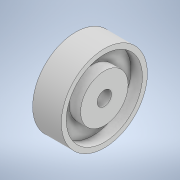
# Autodesk Inventor part: 711145
Saved by Autodesk Inventor 2022 (Build 260153000, 153)
## iProperties
Created: 2021-10-22
Part Number: 711145
Material: Типовые
Document SubType Name: Modeling
Designer: RaNSiD
Density: 1 g/cm^3
Appearance: По умолчанию
Author: RaNSiD
Autodesk Inventor part; units mm, degrees
ref_plane "YZ Plane" through (0, 0, 0) normal (1, 0, 0) x (0, 1, 0)
ref_plane "XZ Plane" through (0, 0, 0) normal (0, 1, 0) x (-1, 0, 0)
ref_plane "XY Plane" through (0, 0, 0) normal (0, 0, 1) x (1, 0, 0)
sketch "Эскиз1" plane through (0, 0, 0) normal (0, 0, 1) x (1, 0, 0)
  line L0 (0, 0) -> (20, 0)
  line L1 (20, 0) -> (20, 30)
  line L2 (20, 30) -> (0, 30)
  line L3 (0, 30) -> (0, 0)
  dimension "d0" = 20
  dimension "d1" = 30
  constraints: 8 end point, 2 parallel, 1 horizontal, 1 perpendicular
  measures "d0" distance of L2.end L1.end
  measures "d1" distance of L1.end L0.end
revolve "Вращение1" add sketch "Эскиз1" angle 360 about axis through (0, 0, 0) along (1, 0, 0)
sketch "Эскиз2" plane through (0, 0, 0) normal (0, 0, 1) x (1, 0, 0)
  line L0 (0, -30) -> (0, 30) projected
  line L1 (0, 15.0882) -> (0, 28)
  line L2 (0, 28) -> (4, 26.5441)
  line L3 (4, 26.5441) -> (4, 16.5441)
  line L4 (4, 16.5441) -> (0, 15.0882)
  line L5 (20, -30) -> (20, 30) projected
  line L6 (20, 26.5441) -> (12, 26.5441)
  line L7 (12, 26.5441) -> (12, 16.5441)
  line L8 (12, 16.5441) -> (20, 16.5441)
  line L9 (20, 16.5441) -> (20, 26.5441)
  line L10 (0, 0) -> (20, 0)
  line L11 (20, 0) -> (20, 5)
  line L12 (20, 5) -> (0, 5)
  line L13 (0, 5) -> (0, 0)
  point P0 (0, 5)
  dimension "d3" = 10
  dimension "d4" = 8
  dimension "d5" = 10
  dimension "d6" = 2
  dimension "d7" = 70
  dimension "d8" = 4
  constraints: 24 end point, 5 parallel, 4 point on line, 2 horizontal, 2 horizontal alignment, 2 perpendicular, 1 equal length
  measures "d3" diameter of L12 L10
  measures "d4" distance of L6.start L6.end
  measures "d5" distance of L6.end L7.end
  measures "d6" distance of L0.end L1.end
  measures "d7" angle of L1 L2
  measures "d8" distance between parallel lines of L1 L3
revolve "Вращение2" cut sketch "Эскиз2" angle 360 about axis through (0, 0, 0) along (1, 0, 0)
